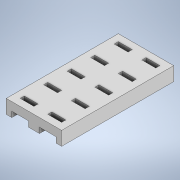
# Autodesk Inventor part: pane_stabilisor
Saved by Autodesk Inventor 2021 (Build 250183000, 183)
## iProperties
Created: 2021-03-18
Part Number: pane_stabilisor
Material: Generisch
Document SubType Name: Modeling
Designer: Tilman
Density: 1 g/cm^3
Appearance: Vorgabe
Author: Tilman
Autodesk Inventor part; units mm, degrees
ref_plane "YZ Plane" through (0, 0, 0) normal (1, 0, 0) x (0, 1, 0)
ref_plane "XZ Plane" through (0, 0, 0) normal (0, 1, 0) x (-1, 0, 0)
ref_plane "XY Plane" through (0, 0, 0) normal (0, 0, 1) x (1, 0, 0)
sketch "Skizze1" plane through (0, 0, 0) normal (0, 1, 0) x (-1, 0, 0)
  line L0 (0, 0) -> (-40, 0)
  line L1 (-40, 0) -> (-40, -81)
  line L2 (-40, -81) -> (0, -81)
  line L3 (0, -81) -> (0, 0)
  line L4 (-5, -8) -> (-15, -8)
  line L5 (-15, -8) -> (-15, -5)
  line L6 (-15, -5) -> (-5, -5)
  line L7 (-5, -5) -> (-5, -8)
  line L8 (-25, -8) -> (-35, -8)
  line L9 (-35, -8) -> (-35, -5)
  line L10 (-35, -5) -> (-25, -5)
  line L11 (-25, -5) -> (-25, -8)
  line L12 (-5, -25) -> (-15, -25)
  line L13 (-15, -25) -> (-15, -22)
  line L14 (-15, -22) -> (-5, -22)
  line L15 (-5, -22) -> (-5, -25)
  line L16 (-25, -25) -> (-35, -25)
  line L17 (-35, -25) -> (-35, -22)
  line L18 (-35, -22) -> (-25, -22)
  line L19 (-25, -22) -> (-25, -25)
  line L20 (-5, -42) -> (-15, -42)
  line L21 (-15, -42) -> (-15, -39)
  line L22 (-15, -39) -> (-5, -39)
  line L23 (-5, -39) -> (-5, -42)
  line L24 (-25, -42) -> (-35, -42)
  line L25 (-35, -42) -> (-35, -39)
  line L26 (-35, -39) -> (-25, -39)
  line L27 (-25, -39) -> (-25, -42)
  line L28 (-5, -59) -> (-15, -59)
  line L29 (-15, -59) -> (-15, -56)
  line L30 (-15, -56) -> (-5, -56)
  line L31 (-5, -56) -> (-5, -59)
  line L32 (-25, -59) -> (-35, -59)
  line L33 (-35, -59) -> (-35, -56)
  line L34 (-35, -56) -> (-25, -56)
  line L35 (-25, -56) -> (-25, -59)
  line L36 (-5, -76) -> (-15, -76)
  line L37 (-15, -76) -> (-15, -73)
  line L38 (-15, -73) -> (-5, -73)
  line L39 (-5, -73) -> (-5, -76)
  line L40 (-25, -76) -> (-35, -76)
  line L41 (-35, -76) -> (-35, -73)
  line L42 (-35, -73) -> (-25, -73)
  line L43 (-25, -73) -> (-25, -76)
  line L44 (-15, -40.5) -> (-25, -40.5) construction
  line L45 (-20, -76) -> (-20, -5) construction
  point P0 (-20, -40.5)
  point P1 (-40, -40.5)
  point P2 (-20, -81)
  dimension "d0" = 3
  dimension "d1" = 10
  dimension "d4" = 20
  dimension "d7" = 17
  dimension "d12" = 5
  dimension "d13" = 5
  constraints: 92 end point, 6 midpoint, 4 parallel, 3 horizontal, 3 horizontal alignment, 2 collinear, 2 perpendicular, 2 vertical, 1 vertical alignment, 70 other
  measures "d0" distance of L4.end L5.end
  measures "d1" distance of L4.start L4.end
  measures "d4" distance of L4.start L8.start
  measures "d7" distance of L4.start L12.start
  measures "d12" distance between parallel lines of L3 L7
  measures "d13" distance between parallel lines of L0 L10
extrude "Extrusion1" add sketch "Skizze1" along normal blind 10
sketch "Skizze2" plane through (0, 0, 0) normal (0, 0, 1) x (1, 0, 0)
  line L0 (0, 0) -> (40, 0) projected
  line L1 (40, 0) -> (40, 10) projected
  line L2 (0, 10) -> (40, 10) projected
  line L3 (0, 0) -> (0, 10) projected
  line L4 (4, 0) -> (4, 4)
  line L5 (4, 4) -> (16, 4)
  line L6 (16, 4) -> (16, 0)
  line L7 (15, 0) -> (5, 0) projected
  line L8 (0, 0) -> (40, 0) projected
  line L9 (24, 0) -> (24, 4)
  line L10 (24, 4) -> (36, 4)
  line L11 (36, 4) -> (36, 0)
  line L12 (35, 0) -> (25, 0) projected
  line L13 (16, 2) -> (24, 2) construction
  point P0 (20, 0)
  point P1 (20, 2)
  point P2 (20, 0)
  dimension "d16" = 4
  dimension "d17" = 12
  dimension "d22" = 8
  constraints: 14 end point, 5 point on line, 4 midpoint, 4 perpendicular, 1 collinear, 1 vertical, 1 vertical alignment, 3 other
  measures "d16" distance of L5.end L6.end
  measures "d17" distance of L4.end L5.end
  measures "d22" distance between parallel lines of L9 L6
extrude "Extrusion2" cut sketch "Skizze2" against normal through all contours L4 L5 L6 L0 | L0 L9 L10 L11
